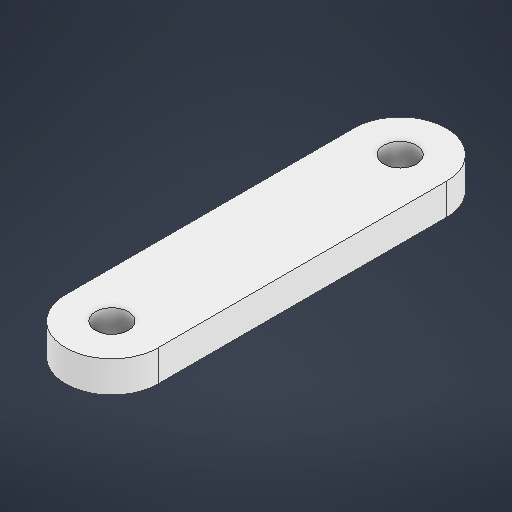
# Autodesk Inventor part: CNC-019-ZAxisBallScrewStabilizerShim2
Saved by Autodesk Inventor 2026.2 (Build 302298000, 298)
## iProperties
Created: 2026-06-22
Part Number: CNC-019-ZAxisBallScrewStabilizerShim2
Material: ABS Plastic
Document SubType Name: Modeling
Designer: Kenji
Density: 1.06 g/cm^3
Appearance: Smooth - White
Author: Kenji
Autodesk Inventor part; units mm, degrees
ref_plane "YZ Plane" through (0, 0, 0) normal (1, 0, 0) x (0, 1, 0)
ref_plane "XZ Plane" through (0, 0, 0) normal (0, 1, 0) x (-1, 0, 0)
ref_plane "XY Plane" through (0, 0, 0) normal (0, 0, 1) x (1, 0, 0)
sketch "Sketch1" plane through (0, 0, 0) normal (0, 1, 0) x (-1, 0, 0)
  circle A0 centre (0, 0) radius 2.6
  circle A1 centre (0, 0) radius 7.3625 construction
  circle A2 centre (0, 46) radius 2.6
  circle A3 centre (0, 46) radius 7.3625 construction
  line L0 (7.3625, 0) -> (7.3625, 46)
  line L1 (-7.3625, 46) -> (-7.3625, 0)
  arc A4 (-7.3625, 0) -> (7.3625, 0) centre (0, 0) ccw
  arc A5 (7.3625, 46) -> (-7.3625, 46) centre (0, 46) ccw
  dimension "d0" = 5.2
  dimension "d1" = 4.7625
  dimension "d2" = 46
  constraints: 8 point on circle, 7 tangent, 6 centre point, 4 end point, 2 coincident, 2 equal radius, 1 vertical alignment
  measures "d0" diameter of A0
  measures "d1" radial gap between concentric circles of A0 A1
  measures "d2" distance of point (0, 0) A2.centre
extrude "Extrusion1" add sketch "Sketch1" along normal blind 5
body "Solid1"
